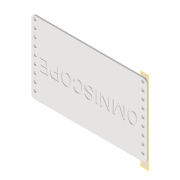
# Autodesk Inventor part: Omniscope_USBC_labellid
Saved by Autodesk Inventor 2022 (Build 260153000, 153)
## iProperties
Created: 2023-05-29
Part Number: Omniscope_USBC_labellid
Material: Generisch
Document SubType Name: Modeling
Designer: diederichbenedict
Density: 1 g/cm^3
Appearance: Vorgabe
Author: diederichbenedict
Autodesk Inventor part; units mm, degrees
ref_plane "YZ Plane" through (0, 0, 0) normal (1, 0, 0) x (0, 1, 0)
ref_plane "XZ Plane" through (0, 0, 0) normal (0, 1, 0) x (-1, 0, 0)
ref_plane "XY Plane" through (0, 0, 0) normal (0, 0, 1) x (1, 0, 0)
ref_plane "Arbeitsebene1" through (0, 0, 0) normal (0, 0, 1) x (1, 0, 0)
sketch "Skizze1" plane through (0, 0, 0) normal (0, 0, 1) x (1, 0, 0)
  line L0 (0, 0) -> (0, -96.9875) projected
  line L1 (-9.5, 0) -> (0, 0) projected
  line L2 (-9.5, 0) -> (-9.5, -87) projected
  arc A0 (-9.5, -87) -> (-4.75, -91.9937) centre (-4.5, -87) ccw projected
  arc A1 (0, -96.9875) -> (-4.75, -91.9937) centre (-5, -96.9875) ccw projected
  circle A2 centre (-5, -84) radius 2 projected
  circle A3 centre (-5, -74) radius 2 projected
  circle A4 centre (-5, -64) radius 2 projected
  circle A5 centre (-5, -54) radius 2 projected
  circle A6 centre (-5, -44) radius 2 projected
  circle A7 centre (-5, -34) radius 2 projected
  circle A8 centre (-5, -24) radius 2 projected
  circle A9 centre (-5, -14) radius 2 projected
  circle A10 centre (-5, -4) radius 2 projected
  arc A11 (-144.092, -92.0063) -> (-139.342, -87.0125) centre (-144.342, -87.0125) ccw projected
  line L3 (-139.342, 0) -> (-139.342, -87.0125) projected
  line L4 (-148.842, 0) -> (-139.342, 0) projected
  line L5 (-148.842, 0) -> (-148.842, -97) projected
  arc A12 (-144.092, -92.0063) -> (-148.842, -97) centre (-143.842, -97) ccw projected
  circle A13 centre (-143.842, -4) radius 2 projected
  circle A14 centre (-143.842, -14) radius 2 projected
  circle A15 centre (-143.842, -24) radius 2 projected
  circle A16 centre (-143.842, -34) radius 2 projected
  circle A17 centre (-143.842, -44) radius 2 projected
  circle A18 centre (-143.842, -54) radius 2 projected
  circle A19 centre (-143.842, -64) radius 2 projected
  circle A20 centre (-143.842, -74) radius 2 projected
  circle A21 centre (-143.842, -84) radius 2 projected
  line L6 (0, 0) -> (-149, 0)
  line L7 (-149, 0) -> (-149, -93.554)
  line L8 (-149, -93.554) -> (0, -93.554)
  line L9 (0, -93.554) -> (0, 0)
  point P0 (-148.842, -93.554)
  dimension "d0" = 149
  constraints: 8 end point, 2 parallel, 1 horizontal, 1 perpendicular
  measures "d0" distance of L8.end L7.end
extrude "Extrusion1" add sketch "Skizze1" along normal blind 2 contours L0 L8 A1 A0 L2 L1 | L2 A0 A1 L8 A12 A11 L3 L6 | L3 A11 A12 L8 L5 L4
fillet "Rundung1" radius 5 4 edges at (0, -93.554, 1) (-148.842, -93.554, 1) (-148.842, 0, 1) (0, 0, 1)
sketch "Skizze2" plane through (0, 0, 2) normal (0, 0, 1) x (1, 0, 0)
  line L0 (-10.6296, -59.1605) -> (-138.3965, -59.1605) construction
  line L1 (-138.3965, -59.1605) -> (-138.3965, -42.7064) construction
  line L2 (-138.3965, -42.7064) -> (-10.6296, -42.7064) construction
  line L3 (-10.6296, -42.7064) -> (-10.6296, -59.1605) construction
  spline S0 degree 2 poles (-24.801, -50.4122) (-24.801, -48.0635) (-23.2176, -44.5537) (-20.3147, -42.7064) (-18.3751, -42.7064) knots 0 0 0 1 2 3 3 3
  spline S1 degree 2 poles (-18.3751, -42.7064) (-16.4882, -42.7064) (-13.5589, -44.5669) (-11.9491, -48.0107) (-11.9227, -50.2671) knots 0 0 0 1 2 3 3 3
  line L4 (-11.9227, -50.2671) -> (-11.9227, -51.4282)
  spline S2 degree 2 poles (-11.9227, -51.4282) (-11.9227, -53.7374) (-13.5325, -57.2736) (-16.4618, -59.1605) (-18.3619, -59.1605) knots 0 0 0 1 2 3 3 3
  spline S3 degree 2 poles (-18.3619, -59.1605) (-20.2751, -59.1605) (-23.2176, -57.3) (-24.801, -53.7769) (-24.801, -51.4282) knots 0 0 0 1 2 3 3 3
  line L5 (-24.801, -51.4282) -> (-24.801, -50.4122)
  spline S4 degree 2 poles (-22.703, -51.4546) (-22.703, -54.3047) (-20.4071, -57.3528) (-18.3619, -57.3528) knots 0 0 0 1 2 2 2
  spline S5 degree 2 poles (-18.3619, -57.3528) (-16.3562, -57.3528) (-14.0603, -54.3047) (-14.0207, -51.5998) knots 0 0 0 1 2 2 2
  line L6 (-14.0207, -51.5998) -> (-14.0207, -50.4254)
  spline S6 degree 2 poles (-14.0207, -50.4254) (-14.0207, -47.6545) (-16.343, -44.5009) (-18.3751, -44.5009) knots 0 0 0 1 2 2 2
  spline S7 degree 2 poles (-18.3751, -44.5009) (-20.4203, -44.5009) (-22.6634, -47.4829) (-22.703, -50.2671) knots 0 0 0 1 2 2 2
  line L7 (-22.703, -50.2671) -> (-22.703, -51.4546)
  line L8 (-30.686, -58.9362) -> (-35.9244, -45.8732)
  line L9 (-35.9244, -45.8732) -> (-41.1496, -58.9362)
  line L10 (-41.1496, -58.9362) -> (-43.8941, -58.9362)
  line L11 (-43.8941, -58.9362) -> (-43.8941, -42.9307)
  line L12 (-43.8941, -42.9307) -> (-41.7829, -42.9307)
  line L13 (-41.7829, -42.9307) -> (-41.7829, -49.1587)
  line L14 (-41.7829, -49.1587) -> (-41.9809, -55.8881)
  line L15 (-41.9809, -55.8881) -> (-36.7293, -42.9307)
  line L16 (-36.7293, -42.9307) -> (-35.1063, -42.9307)
  line L17 (-35.1063, -42.9307) -> (-29.8679, -55.8618)
  line L18 (-29.8679, -55.8618) -> (-30.079, -49.1587)
  line L19 (-30.079, -49.1587) -> (-30.079, -42.9307)
  line L20 (-30.079, -42.9307) -> (-27.9678, -42.9307)
  line L21 (-27.9678, -42.9307) -> (-27.9678, -58.9362)
  line L22 (-27.9678, -58.9362) -> (-30.686, -58.9362)
  line L23 (-59.9128, -42.9307) -> (-57.7884, -42.9307)
  line L24 (-57.7884, -42.9307) -> (-49.7263, -55.268)
  line L25 (-49.7263, -55.268) -> (-49.7263, -42.9307)
  line L26 (-49.7263, -42.9307) -> (-47.6151, -42.9307)
  line L27 (-47.6151, -42.9307) -> (-47.6151, -58.9362)
  line L28 (-47.6151, -58.9362) -> (-49.7263, -58.9362)
  line L29 (-49.7263, -58.9362) -> (-57.8148, -46.5461)
  line L30 (-57.8148, -46.5461) -> (-57.8148, -58.9362)
  line L31 (-57.8148, -58.9362) -> (-59.9128, -58.9362)
  line L32 (-59.9128, -58.9362) -> (-59.9128, -42.9307)
  line L33 (-65.9165, -42.9307) -> (-63.8053, -42.9307)
  line L34 (-63.8053, -42.9307) -> (-63.8053, -58.9362)
  line L35 (-63.8053, -58.9362) -> (-65.9165, -58.9362)
  line L36 (-65.9165, -58.9362) -> (-65.9165, -42.9307)
  spline S8 degree 2 poles (-74.4933, -50.0692) (-71.7751, -50.8477) (-69.3076, -53.1172) (-69.3076, -54.793) knots 0 0 0 1 2 2 2
  spline S9 degree 2 poles (-69.3076, -54.793) (-69.3076, -56.6798) (-72.3293, -59.1605) (-74.744, -59.1605) knots 0 0 0 1 2 2 2
  spline S10 degree 2 poles (-74.744, -59.1605) (-76.3933, -59.1605) (-78.9796, -57.8806) (-80.3914, -55.6374) (-80.3914, -54.3179) knots 0 0 0 1 2 3 3 3
  line L37 (-80.3914, -54.3179) -> (-78.2802, -54.3179)
  spline S11 degree 2 poles (-78.2802, -54.3179) (-78.2802, -55.7694) (-76.4329, -57.432) (-74.744, -57.432) knots 0 0 0 1 2 2 2
  spline S12 degree 2 poles (-74.744, -57.432) (-73.187, -57.432) (-71.4452, -56.0597) (-71.4452, -54.8325) knots 0 0 0 1 2 2 2
  spline S13 degree 2 poles (-71.4452, -54.8325) (-71.4452, -53.8561) (-73.0946, -52.497) (-77.0927, -51.3755) (-79.3358, -50.0296) (-80.431, -48.2219) (-80.431, -46.9947) knots 0 0 0 1 2 3 4 5 5 5
  spline S14 degree 2 poles (-80.431, -46.9947) (-80.431, -45.0551) (-77.3962, -42.7064) (-74.8627, -42.7064) knots 0 0 0 1 2 2 2
  spline S15 degree 2 poles (-74.8627, -42.7064) (-73.2133, -42.7064) (-70.35, -43.9731) (-68.8062, -46.1634) (-68.8062, -47.5621) knots 0 0 0 1 2 3 3 3
  line L38 (-68.8062, -47.5621) -> (-70.9174, -47.5621)
  spline S16 degree 2 poles (-70.9174, -47.5621) (-70.9174, -46.1107) (-73.0682, -44.4349) (-74.8627, -44.4349) knots 0 0 0 1 2 2 2
  spline S17 degree 2 poles (-74.8627, -44.4349) (-76.5253, -44.4349) (-78.3066, -45.794) (-78.3066, -48.1559) (-76.6572, -49.4358) (-74.4933, -50.0692) knots 0 0 0 1 2 3 4 4 4
  spline S18 degree 2 poles (-94.9059, -48.0107) (-94.6024, -45.4641) (-91.4488, -42.7064) (-88.8362, -42.7064) knots 0 0 0 1 2 2 2
  spline S19 degree 2 poles (-88.8362, -42.7064) (-85.9993, -42.7064) (-82.5818, -46.7704) (-82.5818, -50.1879) knots 0 0 0 1 2 2 2
  line L39 (-82.5818, -50.1879) -> (-82.5818, -51.7317)
  spline S20 degree 2 poles (-82.5818, -51.7317) (-82.5818, -53.9617) (-84.1784, -57.3396) (-87.1077, -59.1605) (-89.0209, -59.1605) knots 0 0 0 1 2 3 3 3
  spline S21 degree 2 poles (-89.0209, -59.1605) (-91.5807, -59.1605) (-94.6552, -56.3104) (-94.9059, -53.7901) knots 0 0 0 1 2 2 2
  line L40 (-94.9059, -53.7901) -> (-92.7815, -53.7901)
  spline S22 degree 2 poles (-92.7815, -53.7901) (-92.5044, -55.7166) (-90.6703, -57.432) (-89.0209, -57.432) knots 0 0 0 1 2 2 2
  spline S23 degree 2 poles (-89.0209, -57.432) (-87.0021, -57.432) (-84.7062, -54.4367) (-84.7062, -51.6789) knots 0 0 0 1 2 2 2
  line L41 (-84.7062, -51.6789) -> (-84.7062, -50.1219)
  spline S24 degree 2 poles (-84.7062, -50.1219) (-84.7062, -47.5225) (-86.8833, -44.4349) (-88.8362, -44.4349) knots 0 0 0 1 2 2 2
  spline S25 degree 2 poles (-88.8362, -44.4349) (-90.5911, -44.4349) (-92.478, -46.0315) (-92.7815, -48.0107) knots 0 0 0 1 2 2 2
  line L42 (-92.7815, -48.0107) -> (-94.9059, -48.0107)
  spline S26 degree 2 poles (-110.0933, -50.4122) (-110.0933, -48.0635) (-108.5099, -44.5537) (-105.607, -42.7064) (-103.6673, -42.7064) knots 0 0 0 1 2 3 3 3
  spline S27 degree 2 poles (-103.6673, -42.7064) (-101.7805, -42.7064) (-98.8512, -44.5669) (-97.2414, -48.0107) (-97.215, -50.2671) knots 0 0 0 1 2 3 3 3
  line L43 (-97.215, -50.2671) -> (-97.215, -51.4282)
  spline S28 degree 2 poles (-97.215, -51.4282) (-97.215, -53.7374) (-98.8248, -57.2736) (-101.7541, -59.1605) (-103.6541, -59.1605) knots 0 0 0 1 2 3 3 3
  spline S29 degree 2 poles (-103.6541, -59.1605) (-105.5674, -59.1605) (-108.5099, -57.3) (-110.0933, -53.7769) (-110.0933, -51.4282) knots 0 0 0 1 2 3 3 3
  line L44 (-110.0933, -51.4282) -> (-110.0933, -50.4122)
  spline S30 degree 2 poles (-107.9953, -51.4546) (-107.9953, -54.3047) (-105.6994, -57.3528) (-103.6541, -57.3528) knots 0 0 0 1 2 2 2
  spline S31 degree 2 poles (-103.6541, -57.3528) (-101.6485, -57.3528) (-99.3526, -54.3047) (-99.313, -51.5998) knots 0 0 0 1 2 2 2
  line L45 (-99.313, -51.5998) -> (-99.313, -50.4254)
  spline S32 degree 2 poles (-99.313, -50.4254) (-99.313, -47.6545) (-101.6353, -44.5009) (-103.6673, -44.5009) knots 0 0 0 1 2 2 2
  spline S33 degree 2 poles (-103.6673, -44.5009) (-105.7126, -44.5009) (-107.9557, -47.4829) (-107.9953, -50.2671) knots 0 0 0 1 2 2 2
  line L46 (-107.9953, -50.2671) -> (-107.9953, -51.4546)
  line L47 (-115.3713, -49.1983) -> (-115.3713, -42.9307)
  line L48 (-115.3713, -42.9307) -> (-113.2601, -42.9307)
  line L49 (-113.2601, -42.9307) -> (-113.2601, -58.9362)
  line L50 (-113.2601, -58.9362) -> (-119.1582, -58.9362)
  spline S34 degree 2 poles (-119.1582, -58.9362) (-121.784, -58.9362) (-124.7661, -56.2576) (-124.7661, -54.0408) knots 0 0 0 1 2 2 2
  spline S35 degree 2 poles (-124.7661, -54.0408) (-124.7661, -51.7185) (-121.85, -49.1983) (-119.1318, -49.1983) knots 0 0 0 1 2 2 2
  line L51 (-119.1318, -49.1983) -> (-115.3713, -49.1983)
  line L52 (-115.3713, -50.9268) -> (-119.1582, -50.9268)
  spline S36 degree 2 poles (-119.1582, -50.9268) (-120.8472, -50.9268) (-122.6549, -52.5234) (-122.6549, -54.0277) knots 0 0 0 1 2 2 2
  spline S37 degree 2 poles (-122.6549, -54.0277) (-122.6549, -55.4527) (-120.8472, -57.1812) (-119.277, -57.2076) knots 0 0 0 1 2 2 2
  line L53 (-119.277, -57.2076) -> (-115.3713, -57.2076)
  line L54 (-115.3713, -57.2076) -> (-115.3713, -50.9268)
  line L55 (-136.4964, -50.3199) -> (-129.5691, -50.3199)
  line L56 (-129.5691, -50.3199) -> (-129.5691, -44.6592)
  line L57 (-129.5691, -44.6592) -> (-137.618, -44.6592)
  line L58 (-137.618, -44.6592) -> (-137.618, -42.9307)
  line L59 (-137.618, -42.9307) -> (-127.4579, -42.9307)
  line L60 (-127.4579, -42.9307) -> (-127.4579, -58.9362)
  line L61 (-127.4579, -58.9362) -> (-137.5124, -58.9362)
  line L62 (-137.5124, -58.9362) -> (-137.5124, -57.2076)
  line L63 (-137.5124, -57.2076) -> (-129.5691, -57.2076)
  line L64 (-129.5691, -57.2076) -> (-129.5691, -52.0484)
  line L65 (-129.5691, -52.0484) -> (-136.4964, -52.0484)
  line L66 (-136.4964, -52.0484) -> (-136.4964, -50.3199)
  point P0 (0, 0)
  constraints: 2 other
extrude "Extrusion2" cut sketch "Skizze2" against normal blind 1
